Autodesk Fusion 360 part; units mm, degrees
(part 2 of 5)
sketch "Sketch2" plane through (0, 0, 2) normal (0, 0, 1) x (1, 0, 0)
  arc A0 (2.7973, 14.2208) -> (-2.7973, 14.2208) centre (0, 7.804) ccw
  line L0 (-2.7973, 14.2208) -> (-10.9121, 10.6832)
  arc A1 (-13.7095, 10.1) -> (-10.9121, 10.6832) centre (-13.7095, 17.1) ccw
  line L1 (-13.7095, 10.1) -> (-14.75, 10.1)
  arc A2 (-14.75, 10.1) -> (-19, 2.4661) centre (-14.75, 5.1) ccw
  arc A3 (-18.55, 0.8857) -> (-19, 2.4661) centre (-21.55, 0.8857) ccw
  line L2 (-18.55, 0.8857) -> (-18.55, -26.4)
  arc A4 (-21.55, -29.4) -> (-18.55, -26.4) centre (-21.55, -26.4) ccw
  line L3 (-21.55, -29.4) -> (-30.5, -29.4)
  arc A5 (-30.5, -29.4) -> (-33.9547, -44.6156) centre (-30.5, -37.4) ccw
  arc A6 (-27.7114, -50.1961) -> (-33.9547, -44.6156) centre (-40.4322, -58.1449) ccw
  line L4 (-27.7114, -50.1961) -> (-23.2215, -57.3816)
  arc A7 (-21.55, -63.2107) -> (-23.2215, -57.3816) centre (-32.55, -63.2107) ccw
  line L5 (-21.55, -63.2107) -> (-21.55, -94.9296)
  arc A8 (-23.2215, -100.7587) -> (-21.55, -94.9296) centre (-32.55, -94.9296) ccw
  line L6 (-23.2215, -100.7587) -> (-29.5877, -110.9469)
  arc A9 (-31.6483, -113.6894) -> (-29.5877, -110.9469) centre (-46.5487, -100.3485) ccw
  line L7 (-31.6483, -113.6894) -> (-36.4601, -119.0636)
  arc A10 (-36.4601, -119.0636) -> (-27.3521, -131.7546) centre (-30.5, -124.4) ccw
  line L8 (-27.3521, -131.7546) -> (-8.3, -123.6)
  arc A11 (-4.5, -123.6) -> (-8.3, -123.6) centre (-6.4, -126.96) ccw
  line L9 (-4.5, -123.6) -> (4.5, -123.6)
  arc A12 (8.3, -123.6) -> (4.5, -123.6) centre (6.4, -126.96) ccw
  line L10 (8.3, -123.6) -> (27.3521, -131.7546)
  arc A13 (27.3521, -131.7546) -> (36.4601, -119.0636) centre (30.5, -124.4) ccw
  line L11 (36.4601, -119.0636) -> (31.6483, -113.6894)
  arc A14 (29.5877, -110.9469) -> (31.6483, -113.6894) centre (46.5487, -100.3485) ccw
  line L12 (29.5877, -110.9469) -> (23.2215, -100.7587)
  arc A15 (21.55, -94.9296) -> (23.2215, -100.7587) centre (32.55, -94.9296) ccw
  line L13 (21.55, -94.9296) -> (21.55, -63.2107)
  arc A16 (23.2215, -57.3816) -> (21.55, -63.2107) centre (32.55, -63.2107) ccw
  line L14 (23.2215, -57.3816) -> (27.7114, -50.1961)
  arc A17 (33.9547, -44.6156) -> (27.7114, -50.1961) centre (40.4322, -58.1449) ccw
  arc A18 (33.9547, -44.6156) -> (30.5, -29.4) centre (30.5, -37.4) ccw
  line L15 (30.5, -29.4) -> (21.55, -29.4)
  arc A19 (18.55, -26.4) -> (21.55, -29.4) centre (21.55, -26.4) ccw
  line L16 (18.55, -26.4) -> (18.55, 0.8857)
  arc A20 (19, 2.4661) -> (18.55, 0.8857) centre (21.55, 0.8857) ccw
  arc A21 (19, 2.4661) -> (14.75, 10.1) centre (14.75, 5.1) ccw
  line L17 (14.75, 10.1) -> (13.7095, 10.1)
  arc A22 (10.9121, 10.6832) -> (13.7095, 10.1) centre (13.7095, 17.1) ccw
  line L18 (10.9121, 10.6832) -> (2.7973, 14.2208)
  circle A23 centre (14.75, 5.1) radius 1.5
  circle A24 centre (15.25, -63.8) radius 2.95
  circle A25 centre (15.25, -35.5) radius 1.5
  circle A26 centre (15.25, -94.3) radius 2.95
  circle A27 centre (30.5, -37.4) radius 2
  circle A28 centre (30.5, -124.4) radius 2
  circle A29 centre (15.25, -108.3) radius 1.5
  circle A30 centre (15, -118.1) radius 2.95
  circle A31 centre (-15.25, -35.5) radius 1.5
  circle A32 centre (-30.5, -37.4) radius 2
  circle A33 centre (-14.75, 5.1) radius 1.5
  circle A34 centre (-15.25, -63.8) radius 2.95
  circle A35 centre (-15.25, -94.3) radius 2.95
  circle A36 centre (-15, -118.1) radius 2.95
  circle A37 centre (-15.25, -108.3) radius 1.5
  circle A38 centre (-30.5, -124.4) radius 2
  line L19 (5.15, -89.2) -> (-5.15, -89.2)
  arc A39 (-7.65, -86.7) -> (-5.15, -89.2) centre (-5.15, -86.7) ccw
  line L20 (-7.65, -86.7) -> (-7.65, -71.4)
  arc A40 (-5.15, -68.9) -> (-7.65, -71.4) centre (-5.15, -71.4) ccw
  line L21 (-5.15, -68.9) -> (5.15, -68.9)
  arc A41 (7.65, -71.4) -> (5.15, -68.9) centre (5.15, -71.4) ccw
  line L22 (7.65, -71.4) -> (7.65, -86.7)
  arc A42 (5.15, -89.2) -> (7.65, -86.7) centre (5.15, -86.7) ccw
  line L23 (5.4482, 6.3017) -> (0.3197, 8.5373)
  arc A43 (0.3197, 8.5373) -> (-0.3197, 8.5373) centre (0, 7.804) ccw
  line L24 (-0.3197, 8.5373) -> (-5.4482, 6.3017)
  line L25 (-1.3481, 1.3661) -> (-5.6227, 4.1031)
  line L26 (0, 26.674) -> (0, -149.1667)
  line L27 (1.3481, 1.3661) -> (5.6227, 4.1031)
  line L28 (13.55, -8.5) -> (13.55, -20.5)
  arc A44 (13.55, -20.5) -> (15.55, -20.5) centre (14.55, -20.5) ccw
  line L29 (15.55, -20.5) -> (15.55, -8.5)
  arc A45 (15.55, -8.5) -> (13.55, -8.5) centre (14.55, -8.5) ccw
  line L30 (14.55, -7.5) -> (14.55, -21.5) construction
  line L31 (18.55, 0.8857) -> (18.55, -26.4)
  circle A46 centre (15.25, -35.5) radius 1.5
  line L32 (9.75, -2.5) -> (9.75, -14.5)
  arc A47 (9.75, -14.5) -> (11.75, -14.5) centre (10.75, -14.5) ccw
  line L33 (11.75, -14.5) -> (11.75, -2.5)
  arc A48 (11.75, -2.5) -> (9.75, -2.5) centre (10.75, -2.5) ccw
  line L34 (10.75, -1.5) -> (10.75, -15.5) construction
  line L35 (2.35, -6.7029) -> (2.35, -10.5206)
  line L36 (7.55, -4.3629) -> (7.55, -11.0338)
  line L37 (3.3637, -4.8501) -> (5.7029, -3.3523)
  line L38 (3.3622, -12.3724) -> (4.1622, -12.8855)
  arc A49 (3.3637, -4.8501) -> (2.35, -6.7029) centre (4.55, -6.7029) ccw
  arc A50 (2.35, -10.5206) -> (3.3622, -12.3724) centre (4.55, -10.5206) ccw
  arc A51 (4.1622, -12.8855) -> (7.55, -11.0338) centre (5.35, -11.0338) ccw
  arc A52 (7.55, -4.3629) -> (5.7029, -3.3523) centre (6.35, -4.3629) ccw
  line L39 (2.35, -19.8578) -> (2.35, -23.0931)
  line L40 (9.65, -23.8089) -> (9.65, -25.2396)
  line L41 (4.253, -18.8853) -> (8.8217, -22.188)
  line L42 (2.818, -24.044) -> (6.43, -26.8244)
  arc A53 (4.253, -18.8853) -> (2.35, -19.8578) centre (3.55, -19.8578) ccw
  arc A54 (2.35, -23.0931) -> (2.818, -24.044) centre (3.55, -23.0931) ccw
  arc A55 (6.43, -26.8244) -> (9.65, -25.2396) centre (7.65, -25.2396) ccw
  arc A56 (9.65, -23.8089) -> (8.8217, -22.188) centre (7.65, -23.8089) ccw
  arc A57 (-5.4482, 6.3017) -> (-5.6227, 4.1031) centre (-4.9486, 5.1558) ccw
  arc A58 (5.6227, 4.1031) -> (5.4482, 6.3017) centre (4.9486, 5.1558) ccw
  arc A59 (-1.3481, 1.3661) -> (1.3481, 1.3661) centre (0, 3.4715) ccw
  line L43 (-5.15, -68.9) -> (5.15, -68.9)
  line L44 (0, -57.15) -> (6.189, -57.15)
  line L45 (0, -44.45) -> (4.8532, -44.45)
  line L46 (7.8851, -56.2098) -> (15.1961, -44.5098)
  line L47 (7.2976, -57.15) -> (28.8558, -57.15) construction
  line L48 (10.3384, -41.45) -> (13.5, -41.45)
  line L49 (4.8532, -44.45) -> (6.0958, -43.2074)
  line L50 (4.8532, -44.45) -> (9.5326, -44.45) construction
  arc A60 (10.3384, -41.45) -> (6.0958, -43.2074) centre (10.3384, -47.45) ccw
  arc A61 (15.1961, -44.5098) -> (13.5, -41.45) centre (13.5, -43.45) ccw
  arc A62 (6.189, -57.15) -> (7.8851, -56.2098) centre (6.189, -55.15) ccw
  line L51 (0, -100.95) -> (6.6112, -100.95)
  line L52 (0, -105.45) -> (4.5, -105.45)
  line L53 (4.5, -123.6) -> (4.5, -105.45) construction
  line L54 (8.0447, -101.6962) -> (8.3897, -102.1889)
  line L55 (7.5222, -100.95) -> (12.5593, -100.95) construction
  arc A63 (4.5, -105.45) -> (8.3897, -102.1889) centre (6.3028, -103.6501) ccw
  arc A64 (8.0447, -101.6962) -> (6.6112, -100.95) centre (6.6112, -102.7) ccw
  line L56 (0, -105.45) -> (-4.5, -105.45)
  line L57 (-8.0447, -101.6962) -> (-8.3897, -102.1889)
  arc A65 (-8.3897, -102.1889) -> (-4.5, -105.45) centre (-6.3028, -103.6501) ccw
  arc A66 (-6.6112, -100.95) -> (-8.0447, -101.6962) centre (-6.6112, -102.7) ccw
  line L58 (0, -100.95) -> (-6.6112, -100.95)
  line L59 (0, -44.45) -> (-4.8532, -44.45)
  arc A67 (-6.0958, -43.2074) -> (-10.3384, -41.45) centre (-10.3384, -47.45) ccw
  line L60 (-7.8851, -56.2098) -> (-15.1961, -44.5098)
  line L61 (-10.3384, -41.45) -> (-13.5, -41.45)
  line L62 (0, -57.15) -> (-6.189, -57.15)
  line L63 (-4.8532, -44.45) -> (-9.5326, -44.45) construction
  arc A68 (-7.8851, -56.2098) -> (-6.189, -57.15) centre (-6.189, -55.15) ccw
  line L64 (-4.8532, -44.45) -> (-6.0958, -43.2074)
  arc A69 (-13.5, -41.45) -> (-15.1961, -44.5098) centre (-13.5, -43.45) ccw
  arc A70 (-5.7029, -3.3523) -> (-7.55, -4.3629) centre (-6.35, -4.3629) ccw
  arc A71 (-13.55, -8.5) -> (-15.55, -8.5) centre (-14.55, -8.5) ccw
  arc A72 (-8.8217, -22.188) -> (-9.65, -23.8089) centre (-7.65, -23.8089) ccw
  arc A73 (-9.65, -25.2396) -> (-6.43, -26.8244) centre (-7.65, -25.2396) ccw
  line L65 (-9.65, -23.8089) -> (-9.65, -25.2396)
  line L66 (-13.55, -8.5) -> (-13.55, -20.5)
  line L67 (-3.3637, -4.8501) -> (-5.7029, -3.3523)
  arc A74 (-15.55, -20.5) -> (-13.55, -20.5) centre (-14.55, -20.5) ccw
  arc A75 (-7.55, -11.0338) -> (-4.1622, -12.8855) centre (-5.35, -11.0338) ccw
  arc A76 (-3.3622, -12.3724) -> (-2.35, -10.5206) centre (-4.55, -10.5206) ccw
  line L68 (-15.55, -20.5) -> (-15.55, -8.5)
  line L69 (-10.75, -1.5) -> (-10.75, -15.5) construction
  line L70 (-4.253, -18.8853) -> (-8.8217, -22.188)
  line L71 (-14.55, -7.5) -> (-14.55, -21.5) construction
  line L72 (-2.818, -24.044) -> (-6.43, -26.8244)
  line L73 (-2.35, -19.8578) -> (-2.35, -23.0931)
  line L74 (-2.35, -6.7029) -> (-2.35, -10.5206)
  arc A77 (-2.35, -19.8578) -> (-4.253, -18.8853) centre (-3.55, -19.8578) ccw
  line L75 (-7.55, -4.3629) -> (-7.55, -11.0338)
  line L76 (-9.75, -2.5) -> (-9.75, -14.5)
  line L77 (-3.3622, -12.3724) -> (-4.1622, -12.8855)
  line L78 (-11.75, -14.5) -> (-11.75, -2.5)
  arc A78 (-2.35, -6.7029) -> (-3.3637, -4.8501) centre (-4.55, -6.7029) ccw
  arc A79 (-11.75, -14.5) -> (-9.75, -14.5) centre (-10.75, -14.5) ccw
  arc A80 (-9.75, -2.5) -> (-11.75, -2.5) centre (-10.75, -2.5) ccw
  arc A81 (-2.818, -24.044) -> (-2.35, -23.0931) centre (-3.55, -23.0931) ccw
  point P0 (15.25, -35.5)
  point P1 (-7.5222, -100.95)
  point P2 (-7.2976, -57.15)
  point P3 (-18.55, -26.4)
  point P4 (-18.55, -26.4)
  dimension "d55" = 2
  dimension "d56" = 14
  dimension "d57" = 3
  dimension "d58" = 14
  dimension "d59" = 2
  dimension "d60" = 14
  dimension "d61" = 1.8
  dimension "d62" = 6
  dimension "d63" = 2.35
  dimension "d64" = 5.2
  dimension "d65" = 2.2
  dimension "d66" = 1.2
  dimension "d67" = 2.35
  dimension "d68" = 7.3
  dimension "d69" = 1.2
  dimension "d70" = 2
  dimension "d71" = 1.25
  dimension "d72" = 1.25
  dimension "d73" = 2.5
  dimension "d74" = 11.75
  dimension "d75" = 12.7
  dimension "d76" = 58
  dimension "d77" = 3
  dimension "d78" = 45
  dimension "d79" = 6
  dimension "d80" = 2
  dimension "d81" = 2
  dimension "d82" = 11.75
  dimension "d83" = 4.5
  dimension "d84" = 55
  dimension "d85" = 1.75
  dimension "d86" = 13.5
  constraint tangent L28 A44
  constraint tangent A44 L29
  constraint parallel L28 L29
  constraint tangent L29 A45
  constraint tangent L28 A45
  constraint midpoint A45 L30.start
  constraint midpoint A44 L30.end
  constraint vertical L30
  constraint tangent L32 A47
  constraint tangent A47 L33
  constraint parallel L32 L33
  constraint tangent L33 A48
  constraint tangent L32 A48
  constraint midpoint A48 L34.start
  constraint midpoint A47 L34.end
  constraint vertical L34
  constraint parallel L32 L35
  constraint parallel L34 L36
  constraint parallel L27 L37
  constraint tangent L37 A49
  constraint tangent L35 A49
  constraint tangent L35 A50
  constraint tangent L38 A50
  constraint equal A49 A50
  constraint tangent L38 A51
  constraint tangent L36 A51
  constraint equal A49 A51
  constraint tangent L37 A52
  constraint tangent L36 A52
  constraint vertical L39
  constraint vertical L40
  constraint tangent L41 A53
  constraint tangent L39 A53
  constraint tangent L42 A54
  constraint tangent L39 A54
  constraint equal A53 A54
  constraint tangent L42 A55
  constraint tangent L40 A55
  constraint tangent L40 A56
  constraint tangent L41 A56
  constraint equal A55 A56
  constraint concentric A0 A43
  constraint tangent L23 A43
  constraint tangent A43 L24
  constraint tangent L25 A57
  constraint tangent L24 A57
  constraint tangent L23 A58
  constraint tangent L27 A58
  constraint tangent L27 A59
  constraint tangent L25 A59
  constraint coincident L26 L44.start
  constraint perpendicular L26 L44
  constraint coincident L26 L45.start
  constraint perpendicular L26 L45
  constraint horizontal L47
  constraint horizontal L48
  constraint horizontal L50
  constraint tangent L48 A60
  constraint tangent L49 A60
  constraint tangent L46 A61
  constraint tangent L48 A61
  constraint coincident L47.start L46
  constraint coincident L47.start L44
  constraint tangent L46 A62
  constraint tangent L44 A62
  constraint coincident L26 L51.start
  constraint perpendicular L26 L51
  constraint coincident L26 L52.start
  constraint perpendicular L26 L52
  constraint coincident L9.end A12.end
  constraint vertical L53
  constraint horizontal L55
  constraint tangent L54 A63
  constraint coincident L55.start L54
  constraint coincident L55.start L51
  constraint tangent L54 A64
  constraint tangent L51 A64
  constraint symmetric L26 L51.start L58.start
  constraint symmetric L26 L55.start P1
  constraint symmetric L26 L52.start L56.start
  constraint symmetric L26 L52.end L56.end
  constraint symmetric L26 L54.end L57.end
  constraint symmetric L26 A63 A65
  constraint symmetric L26 L54.start L57.start
  constraint symmetric L26 L51.end A66.start
  constraint symmetric L26 A64 A66
  constraint symmetric L26 L44.start L62.start
  constraint symmetric L26 L47.start P2
  constraint symmetric L26 L45.start L59.start
  constraint symmetric L26 L45.end L59.end
  constraint symmetric L26 L50.end L63.end
  constraint symmetric L26 L48.start A67.end
  constraint symmetric L26 L49.end A67.start
  constraint symmetric L26 A60 A67
  constraint symmetric L26 L46.end L60.end
  constraint symmetric L26 L48.end L61.end
  constraint symmetric L26 A61 A69
  constraint symmetric L26 L46.start L60.start
  constraint symmetric L26 L44.end L62.end
  constraint symmetric L26 A62 A68
  constraint symmetric A19.start L26 P4
  constraint symmetric L26 L28.start A71.start
  constraint symmetric L26 L28.end L66.end
  constraint symmetric L26 A44.end A74.start
  constraint symmetric L26 L29.end A71.end
  constraint symmetric L26 A44 A74
  constraint symmetric L26 A45 A71
  constraint symmetric L26 L30.start L71.start
  constraint symmetric L26 L30.end L71.end
  constraint symmetric L26 A19.start P4
  constraint symmetric L26 L32.start L76.start
  constraint symmetric L26 L32.end L76.end
  constraint symmetric L26 A47.end L78.start
  constraint symmetric L26 L33.end L78.end
  constraint symmetric L26 A47 A79
  constraint symmetric L26 A48 A80
  constraint symmetric L26 L34.start L69.start
  constraint symmetric L26 L34.end L69.end
  constraint symmetric L26 L37.start L67.start
  constraint symmetric L26 L35.start L74.start
  constraint symmetric L26 A49 A78
  constraint symmetric L26 L35.end A76.end
  constraint symmetric L26 L38.start A76.start
  constraint symmetric L26 A50 A76
  constraint symmetric L26 L38.end A75.end
  constraint symmetric L26 L36.end A75.start
  constraint symmetric L26 A51 A75
  constraint symmetric L26 L37.end A70.start
  constraint symmetric L26 L36.start A70.end
  constraint symmetric L26 A52 A70
  constraint symmetric L26 L41.start L70.start
  constraint symmetric L26 L39.start L73.start
  constraint symmetric L26 A53 A77
  constraint symmetric L26 L42.start L72.start
  constraint symmetric L26 L39.end L73.end
  constraint symmetric L26 A54 A81
  constraint symmetric L26 L42.end A73.end
  constraint symmetric L26 L40.end A73.start
  constraint symmetric L26 A55 A73
  constraint symmetric L26 L40.start A72.end
  constraint symmetric L26 L41.end A72.start
  constraint symmetric L26 A56 A72
  measures "d55" diameter of A44
  measures "d56" distance of L30.start L30.end
  measures "d57" distance of L29 L31
  measures "d58" vertical distance of L30.end P0
  measures "d59" diameter of A47
  measures "d60" distance of L34.start L34.end
  measures "d61" distance of L28 L33
  measures "d62" vertical distance of L30.end L34.end
  measures "d63" distance of L26 L35
  measures "d64" distance of L35 L36
  measures "d65" radius of A49
  measures "d66" radius of A52
  measures "d67" distance of L26 L39
  measures "d68" distance of L39 L40
  measures "d69" radius of A53
  measures "d70" radius of A55
  measures "d71" radius of A57
  measures "d72" radius of A58
  measures "d73" radius of A59
  measures "d74" distance of L43 L44
  measures "d75" distance of L44 L45
  measures "d76" angle of L46 L47
  measures "d77" distance of L45 L48
  measures "d78" angle of L49 L50
  measures "d79" radius of A60
  measures "d80" radius of A61
  measures "d81" radius of A62
  measures "d82" distance of L19 L51
  measures "d83" distance of L51 L52
  measures "d84" angle of L54 L55
  measures "d85" radius of A64
  measures "d86" distance of L26 A61.centre
extrude "Extrude2" cut sketch "Sketch2" against normal blind 2 contours A43 L24 L25 L26 A57 A59 | L23 A43 L26 L27 A58 A59 | L26 L44 L45 L46 L48 L49 A60 A61 A62 | L26 L59 A67 L60 L61 L62 A68 L64 A69 | L26 L51 L52 L54 A63 A64 | L26 L56 L57 A65 A66 L58 | L28 A44 L29 A45 | L32 A47 L33 A48 | L35 L36 L37 L38 A49 A50 A51 A52 | L39 L40 L41 L42 A53 A54 A55 A56 | A70 L67 A75 A76 L74 L75 L77 A78 | A71 L66 A74 L68 | A72 A73 L65 L70 L72 L73 A77 A81 | L76 L78 A79 A80
sketch "Sketch3" plane through (0, 0, 0) normal (0, 0, 1) x (1, 0, 0)
  line L0 (13.55, -20.5) -> (13.55, -8.5)
  arc A0 (15.55, -8.5) -> (13.55, -8.5) centre (14.55, -8.5) ccw
  line L1 (15.55, -8.5) -> (15.55, -20.5)
  arc A1 (13.55, -20.5) -> (15.55, -20.5) centre (14.55, -20.5) ccw
  line L2 (-8.8217, -22.188) -> (-4.253, -18.8853)
  arc A2 (-2.35, -19.8578) -> (-4.253, -18.8853) centre (-3.55, -19.8578) ccw
  line L3 (-2.35, -19.8578) -> (-2.35, -23.0931)
  arc A3 (-2.818, -24.044) -> (-2.35, -23.0931) centre (-3.55, -23.0931) ccw
  line L4 (-2.818, -24.044) -> (-6.43, -26.8244)
  arc A4 (-9.65, -25.2396) -> (-6.43, -26.8244) centre (-7.65, -25.2396) ccw
  line L5 (-9.65, -25.2396) -> (-9.65, -23.8089)
  arc A5 (-8.8217, -22.188) -> (-9.65, -23.8089) centre (-7.65, -23.8089) ccw
  line L6 (5.6227, 4.1031) -> (1.3481, 1.3661)
  arc A6 (-1.3481, 1.3661) -> (1.3481, 1.3661) centre (0, 3.4715) ccw
  line L7 (-1.3481, 1.3661) -> (-5.6227, 4.1031)
  arc A7 (-5.4482, 6.3017) -> (-5.6227, 4.1031) centre (-4.9486, 5.1558) ccw
  line L8 (-5.4482, 6.3017) -> (-0.3197, 8.5373)
  arc A8 (0.3197, 8.5373) -> (-0.3197, 8.5373) centre (0, 7.804) ccw
  line L9 (0.3197, 8.5373) -> (5.4482, 6.3017)
  arc A9 (5.6227, 4.1031) -> (5.4482, 6.3017) centre (4.9486, 5.1558) ccw
  line L10 (-15.55, -20.5) -> (-15.55, -8.5)
  arc A10 (-13.55, -8.5) -> (-15.55, -8.5) centre (-14.55, -8.5) ccw
  line L11 (-13.55, -8.5) -> (-13.55, -20.5)
  arc A11 (-15.55, -20.5) -> (-13.55, -20.5) centre (-14.55, -20.5) ccw
  line L12 (9.75, -14.5) -> (9.75, -2.5)
  arc A12 (11.75, -2.5) -> (9.75, -2.5) centre (10.75, -2.5) ccw
  line L13 (11.75, -2.5) -> (11.75, -14.5)
  arc A13 (9.75, -14.5) -> (11.75, -14.5) centre (10.75, -14.5) ccw
  line L14 (-6.0958, -43.2074) -> (-4.8532, -44.45)
  line L15 (-4.8532, -44.45) -> (4.8532, -44.45)
  line L16 (4.8532, -44.45) -> (6.0958, -43.2074)
  arc A14 (10.3384, -41.45) -> (6.0958, -43.2074) centre (10.3384, -47.45) ccw
  line L17 (10.3384, -41.45) -> (13.5, -41.45)
  arc A15 (15.1961, -44.5098) -> (13.5, -41.45) centre (13.5, -43.45) ccw
  line L18 (15.1961, -44.5098) -> (7.8851, -56.2098)
  arc A16 (6.189, -57.15) -> (7.8851, -56.2098) centre (6.189, -55.15) ccw
  line L19 (6.189, -57.15) -> (-6.189, -57.15)
  arc A17 (-7.8851, -56.2098) -> (-6.189, -57.15) centre (-6.189, -55.15) ccw
  line L20 (-7.8851, -56.2098) -> (-15.1961, -44.5098)
  arc A18 (-13.5, -41.45) -> (-15.1961, -44.5098) centre (-13.5, -43.45) ccw
  line L21 (-13.5, -41.45) -> (-10.3384, -41.45)
  arc A19 (-6.0958, -43.2074) -> (-10.3384, -41.45) centre (-10.3384, -47.45) ccw
  line L22 (2.35, -23.0931) -> (2.35, -19.8578)
  arc A20 (4.253, -18.8853) -> (2.35, -19.8578) centre (3.55, -19.8578) ccw
  line L23 (4.253, -18.8853) -> (8.8217, -22.188)
  arc A21 (9.65, -23.8089) -> (8.8217, -22.188) centre (7.65, -23.8089) ccw
  line L24 (9.65, -23.8089) -> (9.65, -25.2396)
  arc A22 (6.43, -26.8244) -> (9.65, -25.2396) centre (7.65, -25.2396) ccw
  line L25 (6.43, -26.8244) -> (2.818, -24.044)
  arc A23 (2.35, -23.0931) -> (2.818, -24.044) centre (3.55, -23.0931) ccw
  line L26 (-2.35, -6.7029) -> (-2.35, -10.5206)
  arc A24 (-3.3622, -12.3724) -> (-2.35, -10.5206) centre (-4.55, -10.5206) ccw
  line L27 (-3.3622, -12.3724) -> (-4.1622, -12.8855)
  arc A25 (-7.55, -11.0338) -> (-4.1622, -12.8855) centre (-5.35, -11.0338) ccw
  line L28 (-7.55, -11.0338) -> (-7.55, -4.3629)
  arc A26 (-5.7029, -3.3523) -> (-7.55, -4.3629) centre (-6.35, -4.3629) ccw
  line L29 (-5.7029, -3.3523) -> (-3.3637, -4.8501)
  arc A27 (-2.35, -6.7029) -> (-3.3637, -4.8501) centre (-4.55, -6.7029) ccw
  line L30 (-9.75, -2.5) -> (-9.75, -14.5)
  arc A28 (-11.75, -14.5) -> (-9.75, -14.5) centre (-10.75, -14.5) ccw
  line L31 (-11.75, -14.5) -> (-11.75, -2.5)
  arc A29 (-9.75, -2.5) -> (-11.75, -2.5) centre (-10.75, -2.5) ccw
  line L32 (2.35, -10.5206) -> (2.35, -6.7029)
  arc A30 (3.3637, -4.8501) -> (2.35, -6.7029) centre (4.55, -6.7029) ccw
  line L33 (3.3637, -4.8501) -> (5.7029, -3.3523)
  arc A31 (7.55, -4.3629) -> (5.7029, -3.3523) centre (6.35, -4.3629) ccw
  line L34 (7.55, -4.3629) -> (7.55, -11.0338)
  arc A32 (4.1622, -12.8855) -> (7.55, -11.0338) centre (5.35, -11.0338) ccw
  line L35 (4.1622, -12.8855) -> (3.3622, -12.3724)
  arc A33 (2.35, -10.5206) -> (3.3622, -12.3724) centre (4.55, -10.5206) ccw
  line L36 (-6.6112, -100.95) -> (6.6112, -100.95)
  arc A34 (8.0447, -101.6962) -> (6.6112, -100.95) centre (6.6112, -102.7) ccw
  line L37 (8.0447, -101.6962) -> (8.3897, -102.1889)
  arc A35 (4.5, -105.45) -> (8.3897, -102.1889) centre (6.3028, -103.6501) ccw
  line L38 (4.5, -105.45) -> (-4.5, -105.45)
  arc A36 (-8.3897, -102.1889) -> (-4.5, -105.45) centre (-6.3028, -103.6501) ccw
  line L39 (-8.3897, -102.1889) -> (-8.0447, -101.6962)
  arc A37 (-6.6112, -100.95) -> (-8.0447, -101.6962) centre (-6.6112, -102.7) ccw
  arc A38 (2.7973, 14.2208) -> (-2.7973, 14.2208) centre (0, 7.804) ccw
  line L40 (-2.7973, 14.2208) -> (-10.9121, 10.6832)
  arc A39 (-13.7095, 10.1) -> (-10.9121, 10.6832) centre (-13.7095, 17.1) ccw
  line L41 (-13.7095, 10.1) -> (-14.75, 10.1)
  arc A40 (-14.75, 10.1) -> (-19, 2.4661) centre (-14.75, 5.1) ccw
  arc A41 (-18.55, 0.8857) -> (-19, 2.4661) centre (-21.55, 0.8857) ccw
  line L42 (-18.55, 0.8857) -> (-18.55, -26.4)
  arc A42 (-21.55, -29.4) -> (-18.55, -26.4) centre (-21.55, -26.4) ccw
  line L43 (-21.55, -29.4) -> (-30.5, -29.4)
  arc A43 (-30.5, -29.4) -> (-33.9547, -44.6156) centre (-30.5, -37.4) ccw
  arc A44 (-27.7114, -50.1961) -> (-33.9547, -44.6156) centre (-40.4322, -58.1449) ccw
  line L44 (-27.7114, -50.1961) -> (-23.2215, -57.3816)
  arc A45 (-21.55, -63.2107) -> (-23.2215, -57.3816) centre (-32.55, -63.2107) ccw
  line L45 (-21.55, -63.2107) -> (-21.55, -94.9296)
  arc A46 (-23.2215, -100.7587) -> (-21.55, -94.9296) centre (-32.55, -94.9296) ccw
  line L46 (-23.2215, -100.7587) -> (-29.5877, -110.9469)
  arc A47 (-31.6483, -113.6894) -> (-29.5877, -110.9469) centre (-46.5487, -100.3485) ccw
  line L47 (-31.6483, -113.6894) -> (-36.4601, -119.0636)
  arc A48 (-36.4601, -119.0636) -> (-27.3521, -131.7546) centre (-30.5, -124.4) ccw
  line L48 (-27.3521, -131.7546) -> (-8.3, -123.6)
  arc A49 (-4.5, -123.6) -> (-8.3, -123.6) centre (-6.4, -126.96) ccw
  line L49 (-4.5, -123.6) -> (4.5, -123.6)
  arc A50 (8.3, -123.6) -> (4.5, -123.6) centre (6.4, -126.96) ccw
  line L50 (8.3, -123.6) -> (27.3521, -131.7546)
  arc A51 (27.3521, -131.7546) -> (36.4601, -119.0636) centre (30.5, -124.4) ccw
  line L51 (36.4601, -119.0636) -> (31.6483, -113.6894)
  arc A52 (29.5877, -110.9469) -> (31.6483, -113.6894) centre (46.5487, -100.3485) ccw
  line L52 (29.5877, -110.9469) -> (23.2215, -100.7587)
  arc A53 (21.55, -94.9296) -> (23.2215, -100.7587) centre (32.55, -94.9296) ccw
  line L53 (21.55, -94.9296) -> (21.55, -63.2107)
  arc A54 (23.2215, -57.3816) -> (21.55, -63.2107) centre (32.55, -63.2107) ccw
  line L54 (23.2215, -57.3816) -> (27.7114, -50.1961)
  arc A55 (33.9547, -44.6156) -> (27.7114, -50.1961) centre (40.4322, -58.1449) ccw
  arc A56 (33.9547, -44.6156) -> (30.5, -29.4) centre (30.5, -37.4) ccw
  line L55 (30.5, -29.4) -> (21.55, -29.4)
  arc A57 (18.55, -26.4) -> (21.55, -29.4) centre (21.55, -26.4) ccw
  line L56 (18.55, -26.4) -> (18.55, 0.8857)
  arc A58 (19, 2.4661) -> (18.55, 0.8857) centre (21.55, 0.8857) ccw
  arc A59 (19, 2.4661) -> (14.75, 10.1) centre (14.75, 5.1) ccw
  line L57 (14.75, 10.1) -> (13.7095, 10.1)
  arc A60 (10.9121, 10.6832) -> (13.7095, 10.1) centre (13.7095, 17.1) ccw
  line L58 (10.9121, 10.6832) -> (2.7973, 14.2208)
  circle A61 centre (30.5, -37.4) radius 2
  circle A62 centre (15.25, -94.3) radius 2.95
  circle A63 centre (15.25, -63.8) radius 2.95
  circle A64 centre (30.5, -124.4) radius 2
  circle A65 centre (15.25, -35.5) radius 1.5
  circle A66 centre (-30.5, -37.4) radius 2
  circle A67 centre (14.75, 5.1) radius 1.5
  circle A68 centre (-15.25, -108.3) radius 1.5
  circle A69 centre (-15, -118.1) radius 2.95
  circle A70 centre (15.25, -108.3) radius 1.5
  circle A71 centre (-15.25, -94.3) radius 2.95
  circle A72 centre (15, -118.1) radius 2.95
  line L59 (5.15, -89.2) -> (-5.15, -89.2)
  arc A73 (-7.65, -86.7) -> (-5.15, -89.2) centre (-5.15, -86.7) ccw
  line L60 (-7.65, -86.7) -> (-7.65, -71.4)
  arc A74 (-5.15, -68.9) -> (-7.65, -71.4) centre (-5.15, -71.4) ccw
  line L61 (-5.15, -68.9) -> (5.15, -68.9)
  arc A75 (7.65, -71.4) -> (5.15, -68.9) centre (5.15, -71.4) ccw
  line L62 (7.65, -71.4) -> (7.65, -86.7)
  arc A76 (5.15, -89.2) -> (7.65, -86.7) centre (5.15, -86.7) ccw
  circle A77 centre (-30.5, -124.4) radius 2
  circle A78 centre (-15.25, -63.8) radius 2.95
  circle A79 centre (-15.25, -35.5) radius 1.5
  circle A80 centre (-14.75, 5.1) radius 1.5
equation "d11 = ( 29.5 / 2 ) * 1 mm"
equation "d18 = ( 37.1 / 2 ) * 1 mm"
equation "d25 = ( 30.5 / 2 ) * 1 mm"
equation "d33 = ( 43.1 / 2 ) * 1 mm"
equation "d43 = 29.8 mm - 6 mm"
equation "d63 = ( 4.7 / 2 ) * 1 mm"
equation "d67 = d63"
equation "d86 = 15.5 mm - 2 mm"

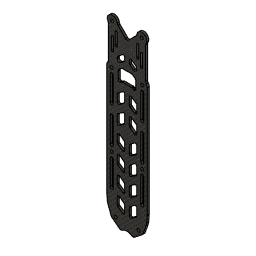
design "top_plate_2mm"
Autodesk Fusion 360 part; units mm, degrees
sketch "Sketch1" plane through (0, 0, 0) normal (0, 0, 1) x (1, 0, 0)
  line L0 (6.189, -57.15) -> (-6.189, -57.15) construction
  arc A0 (33.9547, -44.6156) -> (27.7114, -50.1961) centre (40.4322, -58.1449) ccw construction
  line L1 (-7.8851, -56.2098) -> (-15.1961, -44.5098) construction
  line L2 (15.1961, -44.5098) -> (7.8851, -56.2098) construction
  line L3 (5.15, -89.2) -> (-5.15, -89.2) construction
  arc A1 (6.189, -57.15) -> (7.8851, -56.2098) centre (6.189, -55.15) ccw construction
  arc A2 (-7.8851, -56.2098) -> (-6.189, -57.15) centre (-6.189, -55.15) ccw construction
  arc A3 (-27.7114, -50.1961) -> (-33.9547, -44.6156) centre (-40.4322, -58.1449) ccw construction
  arc A4 (21.55, -94.9296) -> (23.2215, -100.7587) centre (32.55, -94.9296) ccw construction
  line L4 (-5.15, -68.9) -> (5.15, -68.9) construction
  line L5 (21.55, -94.9296) -> (21.55, -63.2107) construction
  line L6 (-7.65, -86.7) -> (-7.65, -71.4) construction
  line L7 (-21.55, -63.2107) -> (-21.55, -94.9296) construction
  line L8 (7.65, -71.4) -> (7.65, -86.7) construction
  line L9 (-27.7114, -50.1961) -> (-23.2215, -57.3816) construction
  arc A5 (-5.15, -68.9) -> (-7.65, -71.4) centre (-5.15, -71.4) ccw construction
  circle A6 centre (15.25, -63.8) radius 2.95 construction
  arc A7 (23.2215, -57.3816) -> (21.55, -63.2107) centre (32.55, -63.2107) ccw construction
  arc A8 (5.15, -89.2) -> (7.65, -86.7) centre (5.15, -86.7) ccw construction
  arc A9 (7.65, -71.4) -> (5.15, -68.9) centre (5.15, -71.4) ccw construction
  arc A10 (-14.75, 10.1) -> (-19, 2.4661) centre (-14.75, 5.1) ccw construction
  arc A11 (-6.0958, -43.2074) -> (-10.3384, -41.45) centre (-10.3384, -47.45) ccw construction
  line L10 (-2.35, -6.7029) -> (-2.35, -10.5206) construction
  arc A12 (8.0447, -101.6962) -> (6.6112, -100.95) centre (6.6112, -102.7) ccw construction
  arc A13 (-5.4482, 6.3017) -> (-5.6227, 4.1031) centre (-4.9486, 5.1558) ccw construction
  line L11 (10.3384, -41.45) -> (13.5, -41.45) construction
  arc A14 (-15.55, -20.5) -> (-13.55, -20.5) centre (-14.55, -20.5) ccw construction
  line L12 (-15.55, -20.5) -> (-15.55, -8.5) construction
  line L13 (-18.55, 0.8857) -> (-18.55, -26.4) construction
  arc A15 (6.43, -26.8244) -> (9.65, -25.2396) centre (7.65, -25.2396) ccw construction
  arc A16 (-4.5, -123.6) -> (-8.3, -123.6) centre (-6.4, -126.96) ccw construction
  line L14 (15.55, -8.5) -> (15.55, -20.5) construction
  arc A17 (-30.5, -29.4) -> (-33.9547, -44.6156) centre (-30.5, -37.4) ccw construction
  line L15 (3.3637, -4.8501) -> (5.7029, -3.3523) construction
  line L16 (-13.7095, 10.1) -> (-14.75, 10.1) construction
  line L17 (8.0447, -101.6962) -> (8.3897, -102.1889) construction
  line L18 (-13.5, -41.45) -> (-10.3384, -41.45) construction
  line L19 (30.5, -29.4) -> (21.55, -29.4) construction
  arc A18 (-11.75, -14.5) -> (-9.75, -14.5) centre (-10.75, -14.5) ccw construction
  line L20 (9.65, -23.8089) -> (9.65, -25.2396) construction
  line L21 (-13.55, -8.5) -> (-13.55, -20.5) construction
  arc A19 (15.1961, -44.5098) -> (13.5, -41.45) centre (13.5, -43.45) ccw construction
  line L22 (13.55, -20.5) -> (13.55, -8.5) construction
  line L23 (-7.55, -11.0338) -> (-7.55, -4.3629) construction
  line L24 (18.55, -26.4) -> (18.55, 0.8857) construction
  arc A20 (-9.65, -25.2396) -> (-6.43, -26.8244) centre (-7.65, -25.2396) ccw construction
  line L25 (-5.7029, -3.3523) -> (-3.3637, -4.8501) construction
  arc A21 (-9.75, -2.5) -> (-11.75, -2.5) centre (-10.75, -2.5) ccw construction
  circle A22 centre (-15.25, -35.5) radius 1.5
  line L26 (-8.8217, -22.188) -> (-4.253, -18.8853) construction
  circle A23 centre (15.25, -108.3) radius 1.5
  line L27 (-31.6483, -113.6894) -> (-36.4601, -119.0636) construction
  line L28 (4.253, -18.8853) -> (8.8217, -22.188) construction
  line L29 (29.5877, -110.9469) -> (23.2215, -100.7587) construction
  line L30 (9.75, -14.5) -> (9.75, -2.5) construction
  circle A24 centre (15, -118.1) radius 2.95 construction
  line L31 (6.43, -26.8244) -> (2.818, -24.044) construction
  arc A25 (-8.3897, -102.1889) -> (-4.5, -105.45) centre (-6.3028, -103.6501) ccw construction
  arc A26 (13.55, -20.5) -> (15.55, -20.5) centre (14.55, -20.5) ccw construction
  line L32 (-21.55, -29.4) -> (-30.5, -29.4) construction
  line L33 (-27.3521, -131.7546) -> (-8.3, -123.6) construction
  line L34 (2.35, -23.0931) -> (2.35, -19.8578) construction
  line L35 (-6.0958, -43.2074) -> (-4.8532, -44.45) construction
  line L36 (-9.65, -25.2396) -> (-9.65, -23.8089) construction
  line L37 (-2.35, -19.8578) -> (-2.35, -23.0931) construction
  line L38 (-11.75, -14.5) -> (-11.75, -2.5) construction
  line L39 (-1.3481, 1.3661) -> (-5.6227, 4.1031) construction
  arc A27 (-7.55, -11.0338) -> (-4.1622, -12.8855) centre (-5.35, -11.0338) ccw construction
  line L40 (-8.3897, -102.1889) -> (-8.0447, -101.6962) construction
  arc A28 (18.55, -26.4) -> (21.55, -29.4) centre (21.55, -26.4) ccw construction
  circle A29 centre (-30.5, -37.4) radius 2 construction
  circle A30 centre (14.75, 5.1) radius 1.5
  circle A31 centre (-14.75, 5.1) radius 1.5
  arc A32 (-13.5, -41.45) -> (-15.1961, -44.5098) centre (-13.5, -43.45) ccw construction
  arc A33 (33.9547, -44.6156) -> (30.5, -29.4) centre (30.5, -37.4) ccw construction
  arc A34 (-5.7029, -3.3523) -> (-7.55, -4.3629) centre (-6.35, -4.3629) ccw construction
  line L41 (4.1622, -12.8855) -> (3.3622, -12.3724) construction
  arc A35 (-2.818, -24.044) -> (-2.35, -23.0931) centre (-3.55, -23.0931) ccw construction
  arc A36 (-3.3622, -12.3724) -> (-2.35, -10.5206) centre (-4.55, -10.5206) ccw construction
  arc A37 (0.3197, 8.5373) -> (-0.3197, 8.5373) centre (0, 7.804) ccw construction
  line L42 (-9.75, -2.5) -> (-9.75, -14.5) construction
  arc A38 (2.35, -10.5206) -> (3.3622, -12.3724) centre (4.55, -10.5206) ccw construction
  line L43 (0.3197, 8.5373) -> (5.4482, 6.3017) construction
  arc A39 (15.55, -8.5) -> (13.55, -8.5) centre (14.55, -8.5) ccw construction
  line L44 (-2.818, -24.044) -> (-6.43, -26.8244) construction
  arc A40 (19, 2.4661) -> (14.75, 10.1) centre (14.75, 5.1) ccw construction
  arc A41 (-8.8217, -22.188) -> (-9.65, -23.8089) centre (-7.65, -23.8089) ccw construction
  arc A42 (-18.55, 0.8857) -> (-19, 2.4661) centre (-21.55, 0.8857) ccw construction
  line L45 (-2.7973, 14.2208) -> (-10.9121, 10.6832) construction
  line L46 (7.55, -4.3629) -> (7.55, -11.0338) construction
  arc A43 (3.3637, -4.8501) -> (2.35, -6.7029) centre (4.55, -6.7029) ccw construction
  arc A44 (11.75, -2.5) -> (9.75, -2.5) centre (10.75, -2.5) ccw construction
  line L47 (11.75, -2.5) -> (11.75, -14.5) construction
  arc A45 (-13.55, -8.5) -> (-15.55, -8.5) centre (-14.55, -8.5) ccw construction
  arc A46 (10.9121, 10.6832) -> (13.7095, 10.1) centre (13.7095, 17.1) ccw construction
  arc A47 (5.6227, 4.1031) -> (5.4482, 6.3017) centre (4.9486, 5.1558) ccw construction
  line L48 (14.75, 10.1) -> (13.7095, 10.1) construction
  line L49 (2.35, -10.5206) -> (2.35, -6.7029) construction
  line L50 (5.6227, 4.1031) -> (1.3481, 1.3661) construction
  arc A48 (9.75, -14.5) -> (11.75, -14.5) centre (10.75, -14.5) ccw construction
  arc A49 (4.1622, -12.8855) -> (7.55, -11.0338) centre (5.35, -11.0338) ccw construction
  arc A50 (7.55, -4.3629) -> (5.7029, -3.3523) centre (6.35, -4.3629) ccw construction
  arc A51 (19, 2.4661) -> (18.55, 0.8857) centre (21.55, 0.8857) ccw construction
  line L51 (-3.3622, -12.3724) -> (-4.1622, -12.8855) construction
  arc A52 (-2.35, -19.8578) -> (-4.253, -18.8853) centre (-3.55, -19.8578) ccw construction
  arc A53 (-2.35, -6.7029) -> (-3.3637, -4.8501) centre (-4.55, -6.7029) ccw construction
  arc A54 (-21.55, -29.4) -> (-18.55, -26.4) centre (-21.55, -26.4) ccw construction
  line L52 (10.9121, 10.6832) -> (2.7973, 14.2208) construction
  arc A55 (-13.7095, 10.1) -> (-10.9121, 10.6832) centre (-13.7095, 17.1) ccw construction
  circle A56 centre (-15.25, -63.8) radius 2.95 construction
  line L53 (4.8532, -44.45) -> (6.0958, -43.2074) construction
  arc A57 (29.5877, -110.9469) -> (31.6483, -113.6894) centre (46.5487, -100.3485) ccw construction
  arc A58 (4.253, -18.8853) -> (2.35, -19.8578) centre (3.55, -19.8578) ccw construction
  arc A59 (10.3384, -41.45) -> (6.0958, -43.2074) centre (10.3384, -47.45) ccw construction
  arc A60 (27.3521, -131.7546) -> (36.4601, -119.0636) centre (30.5, -124.4) ccw construction
  arc A61 (-36.4601, -119.0636) -> (-27.3521, -131.7546) centre (-30.5, -124.4) ccw construction
  circle A62 centre (-15.25, -94.3) radius 2.95 construction
  line L54 (36.4601, -119.0636) -> (31.6483, -113.6894) construction
  arc A63 (4.5, -105.45) -> (8.3897, -102.1889) centre (6.3028, -103.6501) ccw construction
  line L55 (-23.2215, -100.7587) -> (-29.5877, -110.9469) construction
  line L56 (8.3, -123.6) -> (27.3521, -131.7546) construction
  line L57 (-5.4482, 6.3017) -> (-0.3197, 8.5373) construction
  line L58 (4.5, -105.45) -> (-4.5, -105.45) construction
  arc A64 (2.35, -23.0931) -> (2.818, -24.044) centre (3.55, -23.0931) ccw construction
  arc A65 (-1.3481, 1.3661) -> (1.3481, 1.3661) centre (0, 3.4715) ccw construction
  arc A66 (-23.2215, -100.7587) -> (-21.55, -94.9296) centre (-32.55, -94.9296) ccw construction
  line L59 (-6.6112, -100.95) -> (6.6112, -100.95) construction
  circle A67 centre (-30.5, -124.4) radius 2 construction
  line L60 (-4.5, -123.6) -> (4.5, -123.6) construction
  arc A68 (9.65, -23.8089) -> (8.8217, -22.188) centre (7.65, -23.8089) ccw construction
  arc A69 (2.7973, 14.2208) -> (-2.7973, 14.2208) centre (0, 7.804) ccw construction
  circle A70 centre (30.5, -37.4) radius 2 construction
  circle A71 centre (-15.25, -108.3) radius 1.5
  circle A72 centre (-15, -118.1) radius 2.95 construction
  circle A73 centre (30.5, -124.4) radius 2 construction
  arc A74 (-6.6112, -100.95) -> (-8.0447, -101.6962) centre (-6.6112, -102.7) ccw construction
  circle A75 centre (15.25, -94.3) radius 2.95 construction
  circle A76 centre (15.25, -35.5) radius 1.5
  arc A77 (8.3, -123.6) -> (4.5, -123.6) centre (6.4, -126.96) ccw construction
  line L61 (-4.8532, -44.45) -> (4.8532, -44.45) construction
  arc A78 (-31.6483, -113.6894) -> (-29.5877, -110.9469) centre (-46.5487, -100.3485) ccw construction
  line L62 (23.2215, -57.3816) -> (27.7114, -50.1961) construction
  arc A79 (-21.55, -63.2107) -> (-23.2215, -57.3816) centre (-32.55, -63.2107) ccw construction
  arc A80 (-7.65, -86.7) -> (-5.15, -89.2) centre (-5.15, -86.7) ccw construction
  line L63 (21.55, -94.9296) -> (21.55, -63.2107) construction
  line L64 (5.45, -68.479) -> (5.45, -89.621) construction
  circle A81 centre (10, -69.05) radius 1.5 construction
  circle A82 centre (10, -89.05) radius 1.5 construction
  line L65 (-21.55, -63.2107) -> (-21.55, -94.9296) construction
  circle A83 centre (-10, -89.05) radius 1.5 construction
  arc A84 (5.2981, -91.3575) -> (5.45, -89.621) centre (-4.55, -89.621) ccw construction
  arc A85 (5.45, -68.479) -> (5.2981, -66.7425) centre (-4.55, -68.479) ccw construction
  circle A86 centre (30.5, -37.4) radius 3.375 construction
  arc A87 (10.3384, -41.45) -> (6.0958, -43.2074) centre (10.3384, -47.45) ccw construction
  arc A88 (33.9547, -44.6156) -> (27.7114, -50.1961) centre (40.4322, -58.1449) ccw construction
  arc A89 (3.2687, -128.2504) -> (2.5, -129.8265) centre (4.5, -129.8265) ccw construction
  line L66 (5.0629, -146.1617) -> (5.25, -146.1617) construction
  arc A90 (9.1581, -153.5522) -> (8.9013, -150.8916) centre (8.3519, -152.2873) ccw construction
  line L67 (29.5877, -110.9469) -> (23.2215, -100.7587) construction
  arc A91 (22.987, -129.8863) -> (20.2, -131.7249) centre (22.2, -131.7249) ccw construction
  circle A92 centre (-10, -148.1) radius 1 construction
  arc A93 (7.0571, -163.8147) -> (3.1079, -160.45) centre (3.1079, -164.45) ccw construction
  arc A94 (-8.9013, -150.8916) -> (-7, -148.1) centre (-10, -148.1) ccw construction
  arc A95 (9.532, -132.1468) -> (8.688, -130.7979) centre (8.032, -132.1468) ccw construction
  arc A96 (7.3512, -129.5084) -> (8.688, -130.7979) centre (10, -128.1) ccw construction
  line L68 (2.5, -137.5767) -> (2.5, -129.8265) construction
  line L69 (-3.1079, -160.45) -> (3.1079, -160.45) construction
  line L70 (-5.25, -146.1617) -> (-5.0629, -146.1617) construction
  arc A97 (-9.532, -134.0551) -> (-8.8457, -135.3152) centre (-8.032, -134.0551) ccw construction
  line L71 (15.7286, -164.6391) -> (19.1143, -155.3371) construction
  line L72 (-4.1394, -146.4797) -> (-3.0765, -147.3101) construction
  circle A98 centre (-11.5, -163.1) radius 1.5
  arc A99 (29.5877, -110.9469) -> (31.6483, -113.6894) centre (46.5487, -100.3485) ccw construction
  circle A100 centre (-10, -128.1) radius 1 construction
  arc A101 (-15.7286, -164.6391) -> (-7.0571, -163.8147) centre (-11.5, -163.1) ccw construction
  circle A102 centre (11.5, -163.1) radius 1.5
  line L73 (5.2981, -91.3575) -> (4.4577, -96.1236) construction
  arc A103 (-4.0375, -156.816) -> (-2.5, -155.9727) centre (-3.5, -155.9727) ccw construction
  line L74 (7, -147.9117) -> (7, -148.1) construction
  arc A104 (-8.688, -130.7979) -> (-9.532, -132.1468) centre (-8.032, -132.1468) ccw construction
  line L75 (22.987, -129.8863) -> (27.3521, -131.7546) construction
  arc A105 (-2.5, -148.4921) -> (-3.0765, -147.3101) centre (-4, -148.4921) ccw construction
  arc A106 (2.5, -137.5767) -> (4.0425, -138.4168) centre (3.5, -137.5767) ccw construction
  arc A107 (-3.1079, -160.45) -> (-7.0571, -163.8147) centre (-3.1079, -164.45) ccw construction
  circle A108 centre (10, -128.1) radius 1 construction
  arc A109 (19.1143, -155.3371) -> (19.6835, -152.7386) centre (9.7173, -151.9169) ccw construction
  arc A110 (-4.1394, -146.4797) -> (-5.0629, -146.1617) centre (-5.0629, -147.6617) ccw construction
  arc A111 (7, -148.1) -> (8.9013, -150.8916) centre (10, -148.1) ccw construction
  line L76 (19.6835, -152.7386) -> (20.1662, -146.8849) construction
  line L77 (-23.2215, -100.7587) -> (-29.5877, -110.9469) construction
  arc A112 (3.4729, -96.95) -> (4.4577, -96.1236) centre (3.4729, -95.95) ccw construction
  arc A113 (5.0629, -146.1617) -> (4.1394, -146.4797) centre (5.0629, -147.6617) ccw construction
  line L78 (3.4729, -96.95) -> (-3.4729, -96.95) construction
  line L79 (9.1581, -153.5522) -> (4.0375, -156.816) construction
  arc A114 (2.5, -155.9727) -> (4.0375, -156.816) centre (3.5, -155.9727) ccw construction
  line L80 (3.0765, -147.3101) -> (4.1394, -146.4797) construction
  circle A115 centre (15, -148.1) radius 1.5 construction
  line L81 (6.7994, -128.4707) -> (7.3512, -129.5084) construction
  line L82 (9.532, -132.1468) -> (9.532, -134.0551) construction
  arc A116 (7, -147.9117) -> (5.25, -146.1617) centre (5.25, -147.9117) ccw construction
  line L83 (8.8457, -135.3152) -> (4.0425, -138.4168) construction
  circle A117 centre (15.25, -94.3) radius 1.5 construction
  arc A118 (7.0571, -163.8147) -> (15.7286, -164.6391) centre (11.5, -163.1) ccw construction
  line L84 (-7, -148.1) -> (-7, -147.9117) construction
  arc A119 (3.0765, -147.3101) -> (2.5, -148.4921) centre (4, -148.4921) ccw construction
  arc A120 (21.55, -94.9296) -> (23.2215, -100.7587) centre (32.55, -94.9296) ccw construction
  line L85 (4.5, -105.45) -> (-4.5, -105.45) construction
  line L86 (2.5, -155.9727) -> (2.5, -148.4921) construction
  arc A121 (-8.9013, -150.8916) -> (-9.1581, -153.5522) centre (-8.3519, -152.2873) ccw construction
  arc A122 (8.8457, -135.3152) -> (9.532, -134.0551) centre (8.032, -134.0551) ccw construction
  circle A123 centre (30.5, -124.4) radius 3.375 construction
  line L87 (-20.2, -131.7249) -> (-20.2, -146.0632) construction
  line L88 (36.4601, -119.0636) -> (31.6483, -113.6894) construction
  line L89 (-6.6112, -100.95) -> (6.6112, -100.95) construction
  circle A124 centre (15.25, -108.3) radius 1.5 construction
  arc A125 (-3.4729, -61.15) -> (-4.4577, -61.9764) centre (-3.4729, -62.15) ccw construction
  line L90 (8.0447, -101.6962) -> (8.3897, -102.1889) construction
  line L91 (3.2687, -128.2504) -> (3.8022, -127.8336) construction
  circle A126 centre (15, -118.1) radius 1.5 construction
  arc A127 (6.7994, -128.4707) -> (3.8022, -127.8336) centre (5.0335, -129.4096) ccw construction
  line L92 (-3.4729, -61.15) -> (3.4729, -61.15) construction
  line L93 (-4.8532, -44.45) -> (4.8532, -44.45) construction
  arc A128 (4.5, -105.45) -> (8.3897, -102.1889) centre (6.3028, -103.6501) ccw construction
  arc A129 (8.0447, -101.6962) -> (6.6112, -100.95) centre (6.6112, -102.7) ccw construction
  line L94 (6.189, -55.85) -> (-6.189, -55.85) construction
  arc A130 (-21.55, -63.2107) -> (-23.2215, -57.3816) centre (-32.55, -63.2107) ccw construction
  arc A131 (-30.5, -29.4) -> (-33.9547, -44.6156) centre (-30.5, -37.4) ccw construction
  line L95 (20.2, -146.0632) -> (20.2, -131.7249) construction
  arc A132 (27.3521, -131.7546) -> (36.4601, -119.0636) centre (30.5, -124.4) ccw construction
  arc A133 (-36.4601, -119.0636) -> (-27.3521, -131.7546) centre (-30.5, -124.4) ccw construction
  line L96 (-7.3512, -129.5084) -> (-6.7994, -128.4707) construction
  line L97 (-27.3521, -131.7546) -> (-22.987, -129.8863) construction
  circle A134 centre (-15, -118.1) radius 1.5 construction
  arc A135 (20.1662, -146.8849) -> (20.2, -146.0632) centre (10.2, -146.0632) ccw construction
  arc A136 (-19.6835, -152.7386) -> (-19.1143, -155.3371) centre (-9.7173, -151.9169) ccw construction
  circle A137 centre (-15, -148.1) radius 1.5 construction
  arc A138 (-20.2, -146.0632) -> (-20.1662, -146.8849) centre (-10.2, -146.0632) ccw construction
  circle A139 centre (-15.25, -108.3) radius 1.5 construction
  arc A140 (-3.8022, -127.8336) -> (-6.7994, -128.4707) centre (-5.0335, -129.4096) ccw construction
  circle A141 centre (-15.25, -94.3) radius 1.5 construction
  line L98 (-9.532, -134.0551) -> (-9.532, -132.1468) construction
  line L99 (-4.4577, -96.1236) -> (-5.2981, -91.3575) construction
  arc A142 (-20.2, -131.7249) -> (-22.987, -129.8863) centre (-22.2, -131.7249) ccw construction
  arc A143 (-23.2215, -100.7587) -> (-21.55, -94.9296) centre (-32.55, -94.9296) ccw construction
  circle A144 centre (10, -148.1) radius 1 construction
  line L100 (-20.1662, -146.8849) -> (-19.6835, -152.7386) construction
  arc A145 (-31.6483, -113.6894) -> (-29.5877, -110.9469) centre (-46.5487, -100.3485) ccw construction
  circle A146 centre (-30.5, -124.4) radius 3.375 construction
  line L101 (-19.1143, -155.3371) -> (-15.7286, -164.6391) construction
  line L102 (-8.3897, -102.1889) -> (-8.0447, -101.6962) construction
  line L103 (-4.0425, -138.4168) -> (-8.8457, -135.3152) construction
  arc A147 (-6.6112, -100.95) -> (-8.0447, -101.6962) centre (-6.6112, -102.7) ccw construction
  line L104 (-2.5, -148.4921) -> (-2.5, -155.9727) construction
  arc A148 (-4.0425, -138.4168) -> (-2.5, -137.5767) centre (-3.5, -137.5767) ccw construction
  line L105 (-31.6483, -113.6894) -> (-36.4601, -119.0636) construction
  arc A149 (-8.3897, -102.1889) -> (-4.5, -105.45) centre (-6.3028, -103.6501) ccw construction
  arc A150 (-8.688, -130.7979) -> (-7.3512, -129.5084) centre (-10, -128.1) ccw construction
  line L106 (-3.8022, -127.8336) -> (-3.2687, -128.2504) construction
  arc A151 (-4.4577, -96.1236) -> (-3.4729, -96.95) centre (-3.4729, -95.95) ccw construction
  line L107 (-4.0375, -156.816) -> (-9.1581, -153.5522) construction
  arc A152 (-5.25, -146.1617) -> (-7, -147.9117) centre (-5.25, -147.9117) ccw construction
  line L108 (-2.5, -129.8265) -> (-2.5, -137.5767) construction
  arc A153 (-2.5, -129.8265) -> (-3.2687, -128.2504) centre (-4.5, -129.8265) ccw construction
  line L109 (-27.7114, -50.1961) -> (-23.2215, -57.3816) construction
  arc A154 (-6.0958, -43.2074) -> (-10.3384, -41.45) centre (-10.3384, -47.45) ccw construction
  line L110 (-9.313, -29.4) -> (-30.5, -29.4) construction
  arc A155 (-9.313, -29.4) -> (-5, -26.45) centre (-9.313, -24.7722) ccw construction
  arc A156 (-13.5, -41.45) -> (-15.1961, -44.5098) centre (-13.5, -43.45) ccw construction
  line L111 (-9.0119, -54.4991) -> (-15.1961, -44.5098) construction
  line L112 (5, -26.45) -> (-5, -26.45) construction
  circle A157 centre (-30.5, -37.4) radius 3.375 construction
  arc A158 (-27.7114, -50.1961) -> (-33.9547, -44.6156) centre (-40.4322, -58.1449) ccw construction
  circle A159 centre (-10, -69.05) radius 1.5 construction
  spline S0 degree 5 poles (-6.189, -55.85) (-6.3253, -55.85) (-6.5947, -55.8392) (-6.9894, -55.7905) (-7.4965, -55.6656) (-8.0875, -55.414) (-8.5077, -55.1235) (-8.7794, -54.8402) (-8.9382, -54.6183) (-9.0119, -54.4991) knots -1 -1 -1 -1 -1 -1 -0.8 -0.6 -0.4 -0.2 0 0 0 0 0 0 construction
  circle A160 centre (-15.25, -35.5) radius 1.5 construction
  line L113 (-6.0958, -43.2074) -> (-4.8532, -44.45) construction
  line L114 (-13.5, -41.45) -> (-10.3384, -41.45) construction
  line L115 (4.4577, -61.9764) -> (5.2981, -66.7425) construction
  circle A161 centre (15.25, -63.8) radius 1.5 construction
  line L116 (15.1961, -44.5098) -> (9.0119, -54.4991) construction
  circle A162 centre (15.25, -35.5) radius 1.5 construction
  arc A163 (5, -26.45) -> (9.313, -29.4) centre (9.313, -24.7722) ccw construction
  line L117 (10.3384, -41.45) -> (13.5, -41.45) construction
  line L118 (30.5, -29.4) -> (9.313, -29.4) construction
  arc A164 (33.9547, -44.6156) -> (30.5, -29.4) centre (30.5, -37.4) ccw construction
  line L119 (4.8532, -44.45) -> (6.0958, -43.2074) construction
  spline S1 degree 5 poles (9.0119, -54.4991) (8.9382, -54.6183) (8.7794, -54.8402) (8.5077, -55.1235) (8.0875, -55.414) (7.4965, -55.6656) (6.9894, -55.7905) (6.5947, -55.8392) (6.3253, -55.85) (6.189, -55.85) knots 0 0 0 0 0 0 0.2 0.4 0.6 0.8 1 1 1 1 1 1 construction
  line L120 (23.2215, -57.3816) -> (27.7114, -50.1961) construction
  arc A165 (15.1961, -44.5098) -> (13.5, -41.45) centre (13.5, -43.45) ccw construction
  circle A166 centre (-15.25, -63.8) radius 1.5 construction
  line L121 (-5.2981, -66.7425) -> (-4.4577, -61.9764) construction
  arc A167 (23.2215, -57.3816) -> (21.55, -63.2107) centre (32.55, -63.2107) ccw construction
  arc A168 (-5.2981, -66.7425) -> (-5.45, -68.479) centre (4.55, -68.479) ccw construction
  arc A169 (4.4577, -61.9764) -> (3.4729, -61.15) centre (3.4729, -62.15) ccw construction
  line L122 (-5.45, -89.621) -> (-5.45, -68.479) construction
  arc A170 (-5.45, -89.621) -> (-5.2981, -91.3575) centre (4.55, -89.621) ccw construction
  point P0 (0, -44.45)